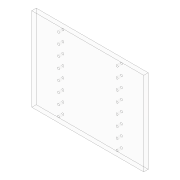
# Autodesk Inventor part: holderStack
Saved by Autodesk Inventor 2018 (Build 220112000, 112)
## iProperties
Created: 2017-05-11
Part Number: holderStack
Material: Polycarbonate, Clear
Document SubType Name: Modeling
Designer: sawaiz
Density: 1.2 g/cm^3
Appearance: Polycarbonate - Clear
Author: sawaiz
Autodesk Inventor part; units mm, degrees
ref_plane "YZ Plane" through (0, 0, 0) normal (1, 0, 0) x (0, 1, 0)
ref_plane "XZ Plane" through (0, 0, 0) normal (0, 1, 0) x (-1, 0, 0)
ref_plane "XY Plane" through (0, 0, 0) normal (0, 0, 1) x (1, 0, 0)
sketch "Sketch1" plane through (0, 0, 0) normal (0, 0, 1) x (1, 0, 0)
  line L0 (-75, -56) -> (75, -56)
  line L1 (75, -56) -> (75, 56)
  line L2 (75, 56) -> (-75, 56)
  line L3 (-75, 56) -> (-75, -56)
  line L4 (-75, -56) -> (75, 56) construction
  line L5 (75, -56) -> (-75, 56) construction
  point P0 (0, 0)
  dimension "d0" = 150
  dimension "d1" = 112
  constraints: 12 end point, 2 midpoint, 2 parallel, 1 horizontal, 1 perpendicular
  measures "d0" distance of L2.end L1.end
  measures "d1" distance of L1.end L0.end
extrude "Extrusion1" add sketch "Sketch1" along normal blind 6
sketch "Sketch2" plane through (0, 0, 6) normal (0, 0, 1) x (1, 0, 0)
  line L0 (-75, -56) -> (75, -56) projected
  line L1 (75, -56) -> (75, 56) projected
  line L2 (75, 56) -> (-75, 56) projected
  line L3 (-75, 56) -> (-75, -56) projected
  line L4 (-39.2, 7) -> (39.2, 7)
  point P0 (0, 0)
  dimension "d4" = 78.4
  dimension "d13" = 7
  dimension "d14" = 39.2
  constraints: 2 end point, 1 horizontal
  measures "d4" distance of L4.start L4.end
  measures "d13" distance from line of point (0, 0) L4
  measures "d14" horizontal distance of point (0, 0) L4.start
hole "Hole1" at (-39.2, 7, 6) at (39.2, 7, 6) direction (0, 0, -1) diameter 2.9 end through all clearance for "Flat Head Machine Screw" size "M2.5" standard "Ansi Metric M Profile"
pattern_linear "Rectangular Pattern1" count 8 spacing 14 along (0, -1, 0) of "Hole1" first direction both ways yes
equation "\"d13\" = 0.5 * tileThickness + 0.5 * tileSeperation"
equation "\"d14\" = 0.5 * d4"
equation "\"d17\" = tileSeperation + tileThickness"
equation "\"tileSeperation\" = 7"
equation "\"tileThickness\" = 7"
body "Solid1"
